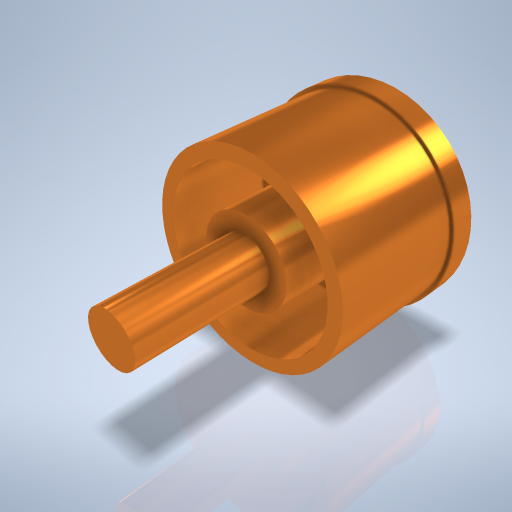
# Autodesk Inventor part: 18
Saved by Autodesk Inventor 2024.2 (Build 282272000, 272)
## iProperties
Created: 2024-05-15
Part Number: 18
Material: Gold
Document SubType Name: Modeling
Designer: Fabri
Density: 19.3 g/cm^3
Appearance: Metall - 1600F (heiß)
Author: Fabri
Autodesk Inventor part; units mm, degrees
ref_plane "XZ Plane" through (0, 0, 0) normal (0, 1, 0) x (-1, 0, 0)
ref_plane "XY Plane" through (0, 0, 0) normal (0, 0, 1) x (1, 0, 0)
sketch "Skizze1" plane through (0, 0, 0) normal (0, 1, 0) x (-1, 0, 0)
  circle A0 centre (0, 0) radius 12.75
  dimension "d0" = 25.5
  constraints: 1 centre point, 1 coincident
  measures "d0" diameter of A0
extrude "Extrusion1" add sketch "Skizze1" along normal blind 3
sketch "Skizze2" plane through (0, 0, 0) normal (0, -1, 0) x (1, 0, 0)
  circle A0 centre (0, 0) radius 12.25
  dimension "d3" = 24.5
  constraints: 1 centre point, 1 coincident
  measures "d3" diameter of A0
extrude "Extrusion2" add sketch "Skizze2" along normal blind 16
sketch "Skizze6" plane through (0, -16, 0) normal (0, -1, 0) x (1, 0, 0)
  circle A0 centre (0, 0) radius 10.5
  dimension "d20" = 21
  constraints: 1 centre point, 1 coincident
  measures "d20" diameter of A0
extrude "Extrusion5" cut sketch "Skizze6" against normal blind 13
sketch "Skizze7" plane through (0, -3, 0) normal (0, -1, 0) x (1, 0, 0)
  circle A0 centre (0, 0) radius 5.5
  dimension "d23" = 11
  constraints: 1 centre point, 1 coincident
  measures "d23" diameter of A0
extrude "Extrusion6" add sketch "Skizze7" along normal up to surface (13 mm away)
sketch "Skizze8" plane through (0, -16, 0) normal (0, -1, 0) x (1, 0, 0)
  circle A0 centre (0, 0) radius 3.25
  dimension "d26" = 6.5
  constraints: 1 centre point, 1 coincident
  measures "d26" diameter of A0
extrude "Extrusion7" add sketch "Skizze8" along normal blind 16
sketch "Skizze9" plane through (0, 3, 0) normal (0, 1, 0) x (1, 0, 0)
  circle A0 centre (0, 0) radius 12.75 projected
  constraints: 1 coincident
hole "Bohrung2" at (0, 3, 0) direction (0, -1, 0) diameter 5 depth 15.8
ref_plane "Arbeitsebene3" through (0, 0, 0) normal (1, 0, 0) x (0, 1, 0)
sketch "Skizze11" plane through (0, 0, 0) normal (1, 0, 0) x (0, 1, 0)
  line L0 (-16, -3.25) -> (-32, -3.25) projected
  line L1 (-3, -5.5) -> (-16, -5.5) projected
  line L2 (-16, -5.5) -> (-16, 5.5) projected
  line L3 (-3, -10.5) -> (-3, 10.5) projected
  line L4 (-30.7422, 0) -> (0, 0)
  line L5 (-22.3, -2) -> (-12.8, -2)
  line L6 (-12.8, -2.5) -> (-12.8, 2.5) projected
  line L7 (-22.3, -2) -> (-22.3, -1.5)
  line L8 (-22.3, -1.5) -> (-28.8, -1.5)
  line L9 (-28.8, -1.5) -> (-28.8, 0)
  line L10 (-12.8, -2) -> (-12.8, 0)
  point P0 (-22.3, -1.75)
  point P1 (-16, -2)
  point P2 (-16, 0)
  dimension "d38" = 3
  dimension "d39" = 4
  dimension "d40" = 9.5
  dimension "d41" = 6.5
  constraints: 12 end point, 3 perpendicular, 2 midpoint, 2 point on line, 1 horizontal, 1 vertical
  measures "d38" diameter of L8 L4
  measures "d39" diameter of L5 L4
  measures "d40" distance from line of point (-22.3, -1.75) L6
  measures "d41" distance between parallel lines of L9 L7
revolve "Umdrehung1" cut sketch "Skizze11" angle 360 about axis through (0, -30.7422, 0) along (0, 1, 0) contours L5 L7 L8 L9 L4 L2
sketch "Skizze14" plane through (0, -12.8, 0) normal (0, 1, 0) x (1, 0, 0)
  point P0 (0, 0)
  point P1 (0, 0)
  constraints: 1 coincident
hole "Bohrung4" at (0, -12.8, 0) direction (0, -1, 0) diameter 4 depth 5
